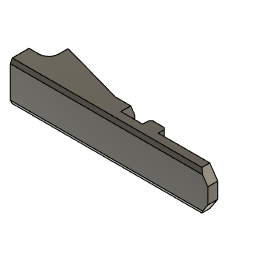
Lead Screw Jig v6 (Autodesk Fusion 360 design; units mm, degrees)
Autodesk Fusion 360 part; units mm, degrees
note: some values were not read from the file. Set by a fixed rule: which sketch regions a step uses.
sketch "Sketch1" plane through (0, 0, 0) normal (0, 0, 1) x (1, 0, 0)
  line L0 (0, 0) -> (0, 7)
  line L1 (0, 0) -> (30, 0)
  line L2 (30, 0) -> (30, -5)
  line L3 (30, -5) -> (-51, -5)
  line L4 (-41.95, 9.5) -> (-41.95, 14.5)
  line L5 (-46, 5.45) -> (-51, 5.45)
  arc A0 (-46, 5.45) -> (-41.95, 9.5) centre (-46, 9.5) ccw
  line L6 (0, 7) -> (-15, 7)
  line L7 (-15, 7) -> (-41.95, 14.5)
  line L8 (-51, 5.45) -> (-51, -5)
  dimension "d1" = 9.5
  dimension "d2" = 46
  dimension "d3" = 8.1
  dimension "d4" = 5
  dimension "d6" = 5
  dimension "d7" = 5
  dimension "d8" = 7
  dimension "d9" = 15
  dimension "d10" = 30
  constraint coincident L0.start L1.start
  constraint vertical L0
  constraint perpendicular L0 L1
  constraint perpendicular L1 L2
  constraint perpendicular L2 L3
  constraint tangent L4 A0
  constraint vertical L4
  constraint tangent L5 A0
  constraint horizontal L5
  constraint perpendicular L0 L6
  constraint perpendicular L5 L8
  measures "d1" distance of L1 A0.centre
  measures "d2" distance of L0 A0.centre
  measures "d3" diameter of A0
  measures "d4" distance of L1.end L2.end
  measures "d6" distance of L5.start L5.end
  measures "d7" distance of L4.start L4.end
  measures "d8" distance of L0.end L1
  measures "d9" distance of L0 L6.end
  measures "d10" distance of L0.start L1.end
extrude "Extrude1" add sketch "Sketch1" along normal blind 20
sketch "Sketch2" plane through (0, -5, 0) normal (0, -1, 0) x (1, 0, 0)
  line L0 (-51, 0) -> (30, 0)
  line L1 (30, 0) -> (30, 20)
  line L2 (30, 20) -> (-51, 20)
  line L3 (15, 20) -> (15, 0) construction
  circle A0 centre (15, 10) radius 3.25
  line L4 (-51, 20) -> (-51, 0)
  dimension "d13" = 15
  dimension "d14" = 6.5
  constraint coincident L2 L3.start
  constraint coincident L0 L3.end
  constraint perpendicular L0 L3
  constraint midpoint L3 A0.centre
  measures "d13" distance of L1 L3
  measures "d14" diameter of A0
chamfer "Chamfer1" distance 1 distance2 2 6 edges at (-43.1362, 6.6362, 20) (-48.5, 5.45, 20) (-41.95, 12, 20) (-43.1362, 6.6362, 0) (-41.95, 12, 0) (-48.5, 5.45, 0) measured on face at (-22, 0.6667, 20) measured on face at (-22, 0.6667, 20) measured on face at (-22, 0.6667, 20) measured on face at (-22, 0.6667, 0) measured on face at (-22, 0.6667, 0) measured on face at (-47.6667, 5.45, 6.6667)
fillet "Fillet1" radius 1 2 edges at (-41.95, 14.5, 10) (-51, 5.45, 10)
chamfer "Chamfer2" distance 4 distance2 6 2 edges at (30, -2.5, 20) (30, -2.5, 0) measured on face at (-22, 0.6667, 20) measured on face at (-22, 0.6667, 0)
chamfer "Chamfer3" distance 1 distance2 2 2 edges at (-12.5, -5, 20) (-12.5, -5, 0) measured on face at (-22, 0.6667, 20) measured on face at (-22, 0.6667, 0)
chamfer "Chamfer4" distance 2 distance2 5 1 edges at (-7.5, 7, 20) measured on face at (-22, 1, 20)
chamfer "Chamfer4" distance 5 distance2 2 1 edges at (-7.5, 7, 0) measured on face at (-5, 7, 6.6667)
sketch "Sketch3" plane through (0, 0, 0) normal (0, 1, 0) x (-1, 0, 0)
  line L0 (-30, 6) -> (-26, 0)
  line L1 (-26, 0) -> (0, 0)
  line L2 (0, 0) -> (0, 20)
  line L3 (0, 20) -> (-26, 20)
  line L4 (-26, 20) -> (-30, 14)
  line L5 (-30, 14) -> (-30, 6)
  line L6 (-18.95, 20) -> (-11.05, 20)
  line L7 (-11.05, 20) -> (-11.05, 0)
  line L8 (-11.05, 0) -> (-18.95, 0)
  line L9 (-18.95, 0) -> (-18.95, 20)
  line L10 (-15, 20) -> (-15, 0) construction
  dimension "d29" = 15
  dimension "d30" = 7.9
  constraint horizontal L6
  constraint vertical L7
  constraint horizontal L8
  constraint vertical L9
  constraint coincident L1 L7.end
  constraint coincident L3 L6.start
  constraint midpoint L6 L10.start
  constraint midpoint L8 L10.end
  measures "d29" distance of L5 L10
  measures "d30" distance of L7 L9
extrude "Extrude3" add sketch "Sketch3" along normal blind 4 contours L1 L3 L6 L7 L8 L9
chamfer "Chamfer5" distance 1 angle 45 2 edges at (18.95, 4, 10) (11.05, 4, 10)
move_face "MoveFace1" by (19, 0, 0) 3 faces at (27.7778, -1.6667, 17.3333) (27.7778, -1.6667, 2.6667) (30, -1.6667, 11.3333)
